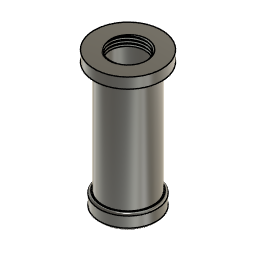
Baloon Sleeve (Autodesk Fusion 360 design; units mm, degrees)
Autodesk Fusion 360 part; units mm, degrees
sketch "Sketch5" plane through (0, 0, 0) normal (0, 0, 1) x (1, 0, 0) in component "Threads on igniter v6"
  line L0 (0, 0) -> (0, 12.7017)
  line L1 (0, 12.7017) -> (11, 6.3509)
  line L2 (11, 6.3509) -> (0, 0)
  line L3 (0, 0) -> (-11, 6.3509)
  line L4 (0, 12.7017) -> (0, 0)
  line L5 (-11, 6.3509) -> (0, 12.7017)
  line L6 (0, 0) -> (-11, -6.3508)
  line L7 (-11, 6.3509) -> (0, 0)
  line L8 (-11, -6.3508) -> (-11, 6.3509)
  line L9 (0, 0) -> (0, -12.7017)
  line L10 (-11, -6.3509) -> (0, 0)
  line L11 (0, -12.7017) -> (-11, -6.3509)
  line L12 (0, 0) -> (11, -6.3509)
  line L13 (0, -12.7017) -> (0, 0)
  line L14 (11, -6.3509) -> (0, -12.7017)
  line L15 (0, 0) -> (11, 6.3508)
  line L16 (11, -6.3509) -> (0, 0)
  line L17 (11, 6.3508) -> (11, -6.3509)
  circle A0 centre (0, 0) radius 16
  dimension "d15" = 12.7017
  dimension "d16" = 60
  dimension "d18" = 360
  dimension "d54" = 32
  constraint coincident L0.start L2.end
  constraint vertical L0
  constraint equal L0 L2
  measures "d15" distance of L0.start L0.end
  measures "d16" angle of L0 L2
  measures "d54" diameter of A0
extrude "Extrude3" add sketch "Sketch5" along normal blind 5 contours L0 L3 L4 L5 L7 | L0 L1 L2 L4 L15 | L3 L6 L7 L8 L10 | L6 L9 L10 L11 L13 | L9 L12 L13 L14 L16 | L2 L12 L15 L16 L17 | A0 in component "Threads on igniter v6"
cylinder "CylinderPrimitive4" cut diameter 18 height -5 placed x (1, 0, 0) y (0, 1, 0) z (0, 0, 1) at (0, 0, 5) in component "Threads on igniter v6"
coil "CoilPrimitive2" add diameter 16.54 section triangle in size 0.92 outside turns 7.0922 pitch 1.41 right hand placed x (1, 0, 0) y (0, 1, 0) z (0, 0, 1) at (0, 0, 0) in component "Threads on igniter v6"
sketch "Sketch14" plane through (0, 0, 5) normal (0, 0, 1) x (-1, 0, 0) in component "Threads on igniter v6"
  arc A0 (-4.4582, -8.0362) -> (-8.1302, 4.2844) centre (0, 0) ccw
  spline S0 degree 3 poles (-4.4582, -8.0362) (-3.3977, -8.5672) (-2.2444, -8.8877) (-0.7611, -8.9989) (-0.4597, -9.0063) (-0.159, -8.9986) knots 0 0 0 0 0.355817 0.355817 0.446405 0.446405 0.446405 0.446405
  arc A1 (-5.0593, 7.4434) -> (-0.159, -8.9986) centre (0, 0) ccw
  circle A2 centre (0, 0) radius 14.7635
  spline S1 degree 3 poles (-5.0593, 7.4434) (-5.2252, 7.3407) (-5.3881, 7.2326) (-6.0701, 6.7468) (-6.5515, 6.3199) (-7.4203, 5.3675) (-7.8044, 4.844) (-8.1302, 4.2844) knots 1.627174 1.627174 1.627174 1.627174 1.685766 1.685766 1.877898 1.877898 2.071762 2.071762 2.071762 2.071762
  circle A3 centre (0, 0) radius 16
  constraint coincident A0.centre A1.centre
extrude "Extrude4" cut sketch "Sketch14" along normal blind 9.5 contours A0 S0 A1 S1 | A2 in component "Threads on igniter v6"
extrude "Extrude5" cut sketch "Sketch5" against normal blind 5 contours L0 L3 L4 L5 L7 | L0 L1 L2 L4 L15 | L3 L6 L7 L8 L10 | L6 L9 L10 L11 L13 | L9 L12 L13 L14 L16 | L2 L12 L15 L16 L17 in component "Threads on igniter v6"
sketch "Sketch18" plane through (0, 0, 5) normal (0, 0, 1) x (-1, 0, 0) in component "Threads on igniter v6"
  arc A0 (-5.0593, 7.4434) -> (-0.159, -8.9986) centre (0, 0) ccw
  spline S0 degree 3 poles (7.9255, 2.3621) (7.7842, 2.9327) (7.5824, 3.4867) (7.0632, 4.5481) (6.7462, 5.0521) (5.6939, 6.3881) (4.8444, 7.1142) (2.8994, 8.2129) (1.8191, 8.5684) (-0.4365, 8.8512) (-1.5908, 8.7685) (-3.5316, 8.2425) (-4.3267, 7.8964) (-5.0593, 7.4434) knots -2.0764 -2.0764 -2.0764 -2.0764 -1.899685 -1.899685 -1.721234 -1.721234 -1.388561 -1.388561 -1.0501 -1.0501 -0.705851 -0.705851 -0.446405 -0.446405 -0.446405 -0.446405
  spline S1 degree 3 poles (-0.159, -8.9986) (0.8069, -8.974) (1.7637, -8.7938) (3.749, -8.0695) (4.7382, -7.4726) (6.4154, -5.9437) (7.0922, -5.0319) (8.0465, -3.0162) (8.3216, -1.9351) (8.4372, 0.2527) (8.284, 1.3376) (7.9255, 2.3621) knots -1.627174 -1.627174 -1.627174 -1.627174 -1.337063 -1.337063 -0.994133 -0.994133 -0.656978 -0.656978 -0.3256 -0.3256 0 0 0 0
  circle A1 centre (0, 0) radius 16
  circle A2 centre (0, 0) radius 9
  line L0 (-5.7895, 6.8907) -> (-3.0727, 8.4592)
  line L1 (-3.0727, 8.4592) -> (-0.4251, 3.8734)
  line L2 (-0.4251, 3.8734) -> (-3.1419, 2.3048)
  line L3 (-3.1419, 2.3048) -> (-5.7895, 6.8907)
  line L4 (0, 0) -> (-4.5, 7.7942)
  dimension "d55" = 18
  constraint concentric A0 A2
  constraint coincident A2 L0.start
  constraint coincident A2 L0.end
  constraint coincident A0.centre A1.centre
  constraint coincident A2 L4.end
  constraint perpendicular L0 L4
  measures "d55" diameter of A2
extrude "Extrude6" cut sketch "Sketch18" against normal up to surface (5 mm away) contours A0 S0 A2 L0 L4 | S0 A2 L4 | L0 L2 L3 L4 | S0 A2 L0 L4 | S0 L0 L4 | S0 L0 L1 L2 L4 | S0 L0 L1 in component "Threads on igniter v6"
sketch "Sketch1" plane through (0, 0, 0) normal (0, 0, -1) x (1, 0, 0)
  arc A0 (9, 0) -> (-2.7226, -8.5783) centre (0, 0) ccw
  line L0 (9, 0) -> (8.27, 0)
  spline S0 degree 3 poles (-2.7226, -8.5783) (-1.7898, -8.8306) (-0.8215, -8.9312) (1.288, -8.8042) (2.4065, -8.5147) (4.4506, -7.5284) (5.3596, -6.8479) (6.8498, -5.1888) (7.4222, -4.2312) (8.1579, -2.1677) (8.321, -1.0841) (8.27, 0) knots -1.627174 -1.627174 -1.627174 -1.627174 -1.337063 -1.337063 -0.994133 -0.994133 -0.656978 -0.656978 -0.3256 -0.3256 0 0 0 0
  circle A1 centre (0, 0) radius 16
  circle A2 centre (0, 0) radius 10
  circle A3 centre (0, 0) radius 12
  dimension "d1" = 24
  constraint concentric A0 A2
  constraint concentric A0 A3
  measures "d1" diameter of A3
extrude "Extrude7" add sketch "Sketch1" along normal blind 60 contours A3 in component "Threads on igniter v6"
sketch "Sketch3" plane through (0, 0, -60) normal (0, 0, -1) x (1, 0, 0)
  circle A0 centre (0, 0) radius 10
  circle A1 centre (0, 0) radius 12
  circle A2 centre (0, 0) radius 13.5
  circle A3 centre (0, 0) radius 8.5
  dimension "d11" = 27
  dimension "d22" = 17
  constraint concentric A0 A2
  constraint concentric A2 A3
  measures "d11" diameter of A2
  measures "d22" diameter of A3
extrude "Extrude9" add sketch "Sketch3" against normal blind 7 contours A2 in component "Threads on igniter v6"
fillet "Fillet3" radius 1 1 edges at (-12.5864, -4.8818, -53) in component "Threads on igniter v6"
fillet "Fillet4" radius 1 1 edges at (-12.5864, 4.8818, -60) in component "Threads on igniter v6"
component "Threads on igniter v6" placed x (1, 0, 0) y (0, 1, 0) z (0, 0, 1) at (0, 0, 0)
equation "d15 = 2 * 11 * 0.57735 mm"
equation "d48 = 10 / 1.41"
